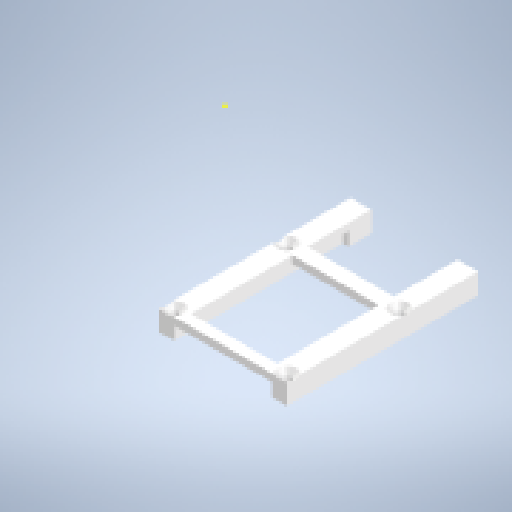
# Autodesk Inventor part: Sliderhalter
Saved by Autodesk Inventor 2025 (Build 290162010, 162A)
## iProperties
Created: 2024-11-26
Part Number: Sliderhalter
Material: PC/ABS-Kunststoff, 3DDruck, PLA
Document SubType Name: Modeling
Designer: Admin
Density: 1.1 g/cm^3
Appearance: Glatt - Weiß(2)
Author: Admin
Autodesk Inventor part; units mm, degrees
ref_plane "YZ Plane" through (0, 0, 0) normal (1, 0, 0) x (0, 1, 0)
ref_plane "XZ Plane" through (0, 0, 0) normal (0, 1, 0) x (-1, 0, 0)
ref_plane "XY Plane" through (0, 0, 0) normal (0, 0, 1) x (1, 0, 0)
sketch "Skizze1" plane through (0, 0, 0) normal (0, 0, 1) x (1, 0, 0)
  line L0 (71.8801, -4.4448) -> (67.8801, -4.4448)
  line L1 (67.8801, -4.4448) -> (67.8801, -55.4448)
  line L2 (67.8801, -55.4448) -> (71.8801, -55.4448)
  line L3 (71.8801, -55.4448) -> (71.8801, -4.4448)
  line L4 (67.8801, -55.4448) -> (41.8801, -55.4448)
  line L5 (41.8801, -55.4448) -> (41.8801, -4.4448)
  line L6 (41.8801, -4.4448) -> (67.8801, -4.4448)
  line L7 (67.8801, -4.4448) -> (67.8801, -55.4448)
  line L8 (41.8801, -55.4448) -> (37.8801, -55.4448)
  line L9 (37.8801, -55.4448) -> (37.8801, -4.4448)
  line L10 (37.8801, -4.4448) -> (41.8801, -4.4448)
  line L11 (41.8801, -4.4448) -> (41.8801, -55.4448)
  point P0 (0, 0)
  dimension "d0" = 4
  dimension "d1" = 51
  dimension "d2" = 26
  dimension "d3" = 4
  constraints: 24 end point, 6 parallel, 3 horizontal, 3 perpendicular, 2 point on line
  measures "d0" distance of L2.end L1.end
  measures "d1" distance of L1.end L0.end
  measures "d2" distance of L5.end L6.end
  measures "d3" distance of L9.end L10.end
extrude "Extrusion1" add sketch "Skizze1" along normal blind 3.5 contours L3 L2 L1 L0 | L5 L8 L9 L10
sketch "Skizze2" plane through (0, 0, 3.5) normal (0, 0, 1) x (1, 0, 0)
  line L0 (71.8801, -55.4448) -> (37.8801, -55.4448)
  line L1 (71.8801, -4.4448) -> (37.8801, -4.4448)
  line L2 (37.8801, -4.4448) -> (37.8801, -55.4448) projected
  line L3 (71.8801, -55.4448) -> (71.8801, -4.4448) projected
  line L4 (43.3801, -4.4448) -> (66.3801, -4.4448)
  line L5 (66.3801, -4.4448) -> (66.3801, -21.4448)
  line L6 (66.3801, -21.4448) -> (43.3801, -21.4448)
  line L7 (43.3801, -21.4448) -> (43.3801, -4.4448)
  line L8 (41.8801, -55.4448) -> (67.8801, -55.4448)
  line L9 (43.3801, -52.4448) -> (66.3801, -52.4448)
  line L10 (66.3801, -52.4448) -> (66.3801, -25.4448)
  line L11 (66.3801, -25.4448) -> (43.3801, -25.4448)
  line L12 (43.3801, -25.4448) -> (43.3801, -52.4448)
  line L13 (41.8801, -55.4448) -> (67.8801, -55.4448)
  line L14 (67.8801, -55.4448) -> (67.8801, -55.4448)
  line L15 (67.8801, -55.4448) -> (41.8801, -55.4448)
  line L16 (41.8801, -55.4448) -> (41.8801, -55.4448)
  point P0 (0, 0)
  point P1 (54.8801, -4.4448)
  point P2 (67.8801, -45.4448)
  point P3 (54.8801, -55.4448)
  dimension "d38" = 23
  dimension "d39" = 17
  dimension "d44" = 4
  dimension "d45" = 0
  dimension "d46" = 3
  dimension "d47" = 26
  constraints: 30 end point, 7 equal length, 5 midpoint, 4 horizontal, 3 perpendicular, 2 collinear, 2 point on line
  measures "d38" distance of L5.end L6.end
  measures "d39" distance of L4.end L5.end
  measures "d44" distance between parallel lines of L6 L11
  measures "d45" distance of L14.end L13.end
  measures "d46" distance between parallel lines of L15 L9
  measures "d47" distance between parallel lines of L14 L16
extrude "Extrusion2" add sketch "Skizze2" along normal blind 2 contours L0 L2 L1 L7 L6 L5 L3
sketch "Skizze3" plane through (0, 0, 5.5) normal (0, 0, 1) x (1, 0, 0)
  line L0 (37.8801, -4.4448) -> (37.8801, -55.4448) projected
  line L1 (39.8801, -23.4448) -> (37.8801, -23.4448) construction
  line L2 (39.8801, -23.4448) -> (41.8801, -23.4448) construction
  line L3 (39.8801, -23.4448) -> (39.8801, -4.4448) construction
  line L4 (69.8801, -23.4448) -> (71.8801, -23.4448) construction
  line L5 (71.8801, -4.4448) -> (37.8801, -4.4448) construction
  line L6 (71.8801, -55.4448) -> (71.8801, -4.4448) projected
  line L7 (71.8801, -55.4448) -> (37.8801, -55.4448)
  line L8 (37.8801, -55.4448) -> (71.8801, -55.4448) projected
  line L9 (39.8801, -53.4448) -> (39.8801, -23.4448)
  line L10 (69.8801, -53.4448) -> (69.8801, -23.4448)
  line L11 (67.8801, -4.4448) -> (67.8801, -55.4448) projected
  line L12 (39.8801, -53.4448) -> (39.8801, -55.4448)
  line L13 (69.8801, -53.4448) -> (69.8801, -55.4448)
  point P0 (0, 0)
  dimension "d24" = 2
  dimension "d37" = 19
  constraints: 18 end point, 10 point on line, 4 equal length, 2 collinear, 2 horizontal, 1 parallel, 1 perpendicular, 1 vertical
  measures "d24" distance of L1.start L1.end
  measures "d37" distance of L1.start L3.end
hole "Bohrung1" at (39.8801, -23.4448, 5.5) at (69.8801, -23.4448, 5.5) at (39.8801, -53.4448, 5.5) at (69.8801, -53.4448, 5.5) direction (0, 0, -1) diameter 2.2 end through all countersink diameter 5 countersink angle 90
sketch "Skizze6" plane through (0, 0, 3.5) normal (0, 0, -1) x (-1, 0, 0)
  line L0 (-67.8801, -4.4448) -> (-67.8801, -55.4448) projected
  line L1 (-66.3801, -4.4448) -> (-66.3801, -21.4448) projected
  line L2 (-67.8801, -4.4448) -> (-66.3801, -4.4448)
  line L3 (-66.3801, -4.4448) -> (-66.3801, -10.4448)
  line L4 (-66.3801, -10.4448) -> (-67.8801, -10.4448)
  line L5 (-67.8801, -10.4448) -> (-67.8801, -4.4448)
  line L6 (-43.3801, -21.4448) -> (-43.3801, -4.4448) projected
  line L7 (-41.8801, -55.4448) -> (-41.8801, -4.4448) projected
  line L8 (-43.3801, -4.4448) -> (-41.8801, -4.4448)
  line L9 (-41.8801, -4.4448) -> (-41.8801, -10.4448)
  line L10 (-41.8801, -10.4448) -> (-43.3801, -10.4448)
  line L11 (-43.3801, -10.4448) -> (-43.3801, -4.4448)
  point P0 (0, 0)
  dimension "d48" = 6
  constraints: 16 end point, 4 parallel, 3 point on line, 2 horizontal, 2 perpendicular
  measures "d48" distance of L2.end L3.end
extrude "Extrusion5" add sketch "Skizze6" along normal up to surface (3.5 mm away)
sketch "Skizze7" plane through (0, 0, 5.5) normal (0, 0, 1) x (1, 0, 0)
  point P0 (0, 0)
